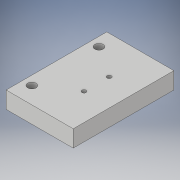
# Autodesk Inventor part: limitSwitchMount
Saved by Autodesk Inventor 2017 (Build 210142000, 142)
## iProperties
Created: 2017-03-20
Part Number: limitSwitchMount
Material: Generic
Document SubType Name: Modeling
Designer: Naga
Density: 1 g/cm^3
Appearance: Default
Author: Naga
Autodesk Inventor part; units mm, degrees
ref_plane "YZ Plane" through (0, 0, 0) normal (1, 0, 0) x (0, 1, 0)
ref_plane "XZ Plane" through (0, 0, 0) normal (0, 1, 0) x (-1, 0, 0)
ref_plane "XY Plane" through (0, 0, 0) normal (0, 0, 1) x (1, 0, 0)
sketch "Sketch1" plane through (0, 0, 0) normal (0, 1, 0) x (-1, 0, 0)
  line L0 (0, 0) -> (25.4, 0)
  line L1 (25.4, 0) -> (25.4, -38.1)
  line L2 (25.4, -38.1) -> (0, -38.1)
  line L3 (0, -38.1) -> (0, 0)
  line L4 (0, -19.05) -> (17.2212, -19.05) construction
  line L5 (17.2212, -19.05) -> (21.9964, -19.05) construction
  line L6 (21.9964, -19.05) -> (21.9964, -31.75) construction
  circle A0 centre (21.9964, -31.75) radius 1.5875
  line L7 (17.2212, -19.05) -> (10.2108, -19.05) construction
  line L8 (10.2108, -19.05) -> (10.2108, -23.8125) construction
  circle A1 centre (10.2108, -23.8125) radius 0.8001
  circle A2 centre (21.9964, -6.35) radius 1.5875
  circle A3 centre (10.2108, -14.2875) radius 0.8001
  dimension "d0" = 25.4
  dimension "d1" = 38.1
  dimension "d2" = 17.2212
  dimension "d3" = 4.7752
  dimension "d4" = 12.7
  dimension "d5" = 3.175
  dimension "d6" = 7.0104
  dimension "d7" = 4.7625
  dimension "d8" = 1.6002
  constraints: 18 end point, 4 centre point, 3 perpendicular, 2 coincident, 2 parallel, 2 point on line, 2 symmetric about line, 1 horizontal, 1 midpoint, 1 vertical, 2 other
  measures "d0" distance of L1.end L2.end
  measures "d1" distance of L0.end L1.end
  measures "d2" distance of L4.start L4.end
  measures "d3" distance of L4.end L5.end
  measures "d4" distance of L5.end L6.end
  measures "d5" diameter of A0
  measures "d6" distance of L4.end L7.end
  measures "d7" distance of L7.end L8.end
  measures "d8" diameter of A1
extrude "Extrusion1" add sketch "Sketch1" along normal blind 6.35
body "Solid1"
